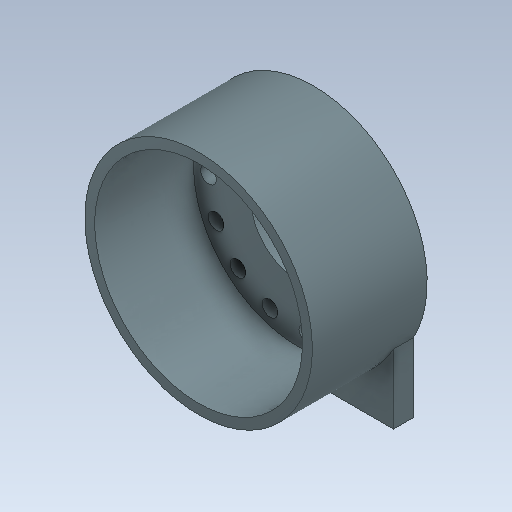
# Autodesk Inventor part: Main Housing
Saved by Autodesk Inventor 2026.2 (Build 302298010, 298A)
## iProperties
Created: 2026-07-17
Part Number: Main Housing
Material: Generic
Document SubType Name: Modeling
Designer: maxim
Density: 1 g/cm^3
Appearance: Lead
Author: maxim
Autodesk Inventor part; units mm, degrees
ref_plane "YZ Plane" through (0, 0, 0) normal (1, 0, 0) x (0, 1, 0)
ref_plane "XZ Plane" through (0, 0, 0) normal (0, 1, 0) x (-1, 0, 0)
ref_plane "XY Plane" through (0, 0, 0) normal (0, 0, 1) x (1, 0, 0)
sketch "Sketch1" plane through (0, 0, 0) normal (0, 0, 1) x (1, 0, 0)
  circle A0 centre (0, 0) radius 52.5
  circle A1 centre (0, 0) radius 57.5
  circle A2 centre (0, 0) radius 23.6
  circle A3 centre (0, 0) radius 21.1
  circle A4 centre (0, 0) radius 45 construction
  line L0 (50.4975, -27.5) -> (50.4975, -62.5)
  line L1 (-50.4975, -27.5) -> (-50.4975, -62.5)
  line L2 (50.4975, -62.5) -> (-50.4975, -62.5)
  line L3 (20.0155, -57.5) -> (-14.9845, -57.5) construction
  circle A5 centre (-45, 0) radius 4
  dimension "d11" = 90
  dimension "d0" = 105
  dimension "d1" = 5
  dimension "d2" = 47.2
  dimension "d3" = 2.5
  dimension "d17" = 35
  dimension "d18" = 35
  dimension "d19" = 5
  dimension "d22" = 8
  constraints: 8 end point, 5 centre point, 3 coincident, 2 horizontal, 2 horizontal alignment, 2 point on circle, 2 vertical, 1 tangent, 2 other
  measures "d0" diameter of A0
  measures "d1" radial gap between concentric circles of A0 A1
  measures "d2" diameter of A2
  measures "d3" radial gap between concentric circles of A2 A3
  measures "d17" distance of L0.start L0.end
  measures "d18" distance of L1.start L1.end
  measures "d19" distance between parallel lines of L2 L3
  measures "d22" diameter of A5
extrude "Extrusion1" add sketch "Sketch1" along normal blind 4 contours A2
extrude "Extrusion2" add sketch "Sketch1" along normal blind 8 contours A0 | A5
extrude "Extrusion3" add sketch "Sketch1" along normal blind 58 contours A1
extrude "Extrusion4" cut sketch "Sketch1" along normal blind 15 contours A5
extrude "Extrusion5" add sketch "Sketch1" along normal blind 10 contours A1 L0 L2 L1
pattern_circular "Circular Pattern2" count 15 over 360 about axis through (0, 0, 0) along (0, 0, 1) of "Extrusion4"
body "Solid1"
